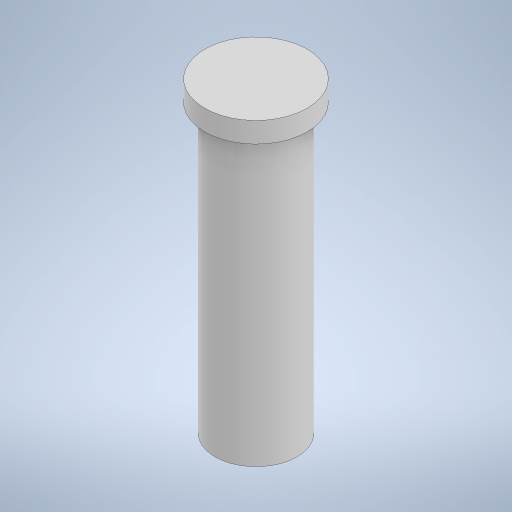
# Autodesk Inventor part: Silander
Saved by Autodesk Inventor 2024 (Build 280153000, 153)
## iProperties
Created: 2024-02-08
Part Number: Silander
Material: Generic
Document SubType Name: Modeling
Designer: yogde
Density: 1 g/cm^3
Appearance: Default
Author: yogde
Autodesk Inventor part; units mm, degrees
ref_plane "YZ Plane" through (0, 0, 0) normal (1, 0, 0) x (0, 1, 0)
ref_plane "XZ Plane" through (0, 0, 0) normal (0, 1, 0) x (-1, 0, 0)
ref_plane "XY Plane" through (0, 0, 0) normal (0, 0, 1) x (1, 0, 0)
sketch "Sketch1" plane through (0, 0, 0) normal (0, 0, 1) x (1, 0, 0)
  line L0 (0, 0) -> (4, 0)
  line L1 (4, 0) -> (4, 28)
  line L2 (4, 28) -> (5, 28)
  line L3 (5, 28) -> (5, 30)
  line L4 (5, 30) -> (0, 30)
  line L5 (0, 30) -> (0, 0)
  dimension "d0" = 4
  dimension "d1" = 28
  dimension "d2" = 1
  dimension "d3" = 2
  dimension "d4" = 5
  constraints: 12 end point, 4 perpendicular, 1 horizontal
  measures "d0" distance of L0.start L0.end
  measures "d1" distance of L0.end L1.end
  measures "d2" distance of L1.end L2.end
  measures "d3" distance of L2.end L3.end
  measures "d4" distance of L3.end L4.end
revolve "Revolution1" add sketch "Sketch1" angle 360 about axis through (0, 30, 0) along (0, -1, 0)
body "Solid1"
